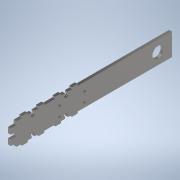
# Autodesk Inventor part: NeckFrame
Saved by Autodesk Inventor 2021 (Build 250183000, 183)
## iProperties
Created: 2021-03-05
Part Number: NeckFrame
Material: Steel, High Strength, Low Alloy
Document SubType Name: Modeling
Designer: M3rob
Density: 7.85 g/cm^3
Appearance: Steel - Polished
Mass: 7033.88 g
Surface Area: 1732.16 cm^2
Volume: 896.036 cm^3
Author: M3rob
Autodesk Inventor part; units mm, degrees
ref_plane "YZ Plane" through (0, 0, 0) normal (1, 0, 0) x (0, 1, 0)
ref_plane "XZ Plane" through (0, 0, 0) normal (0, 1, 0) x (-1, 0, 0)
ref_plane "XY Plane" through (0, 0, 0) normal (0, 0, 1) x (1, 0, 0)
sketch "Sketch1" plane through (0, 0, 0) normal (1, 0, 0) x (0, 1, 0)
  line L0 (50.8, 332.74) -> (34.925, 332.74)
  line L1 (-50.8, 332.74) -> (-50.8, -378.46)
  line L2 (-50.8, -378.46) -> (50.8, -378.46)
  line L3 (50.8, -378.46) -> (50.8, 53.34)
  circle A0 centre (0, -314.96) radius 25.4
  line L4 (50.8, 0) -> (-50.8, 0) construction
  line L5 (50.8, 307.34) -> (58.7375, 307.34)
  line L6 (58.7375, 307.34) -> (58.7375, 281.94)
  line L7 (58.7375, 281.94) -> (50.8, 281.94)
  line L8 (50.8, 281.94) -> (34.925, 281.94) construction
  line L9 (34.925, 281.94) -> (34.925, 307.34) construction
  line L10 (34.925, 307.34) -> (50.8, 307.34) construction
  line L11 (58.7375, 205.74) -> (50.8, 205.74)
  line L12 (58.7375, 231.14) -> (58.7375, 205.74)
  line L13 (50.8, 231.14) -> (58.7375, 231.14)
  line L14 (34.925, 231.14) -> (50.8, 231.14) construction
  line L15 (34.925, 205.74) -> (34.925, 231.14) construction
  line L16 (50.8, 205.74) -> (34.925, 205.74) construction
  line L17 (58.7375, 129.54) -> (50.8, 129.54)
  line L18 (58.7375, 154.94) -> (58.7375, 129.54)
  line L19 (50.8, 154.94) -> (58.7375, 154.94)
  line L20 (34.925, 154.94) -> (50.8, 154.94) construction
  line L21 (34.925, 129.54) -> (34.925, 154.94) construction
  line L22 (50.8, 129.54) -> (34.925, 129.54) construction
  line L23 (58.7375, 53.34) -> (50.8, 53.34)
  line L24 (58.7375, 78.74) -> (58.7375, 53.34)
  line L25 (50.8, 78.74) -> (58.7375, 78.74)
  line L26 (34.925, 78.74) -> (50.8, 78.74) construction
  line L27 (34.925, 53.34) -> (34.925, 78.74) construction
  line L28 (50.8, 53.34) -> (34.925, 53.34) construction
  line L29 (50.8, 281.94) -> (50.8, 307.34) construction
  line L30 (50.8, 307.34) -> (50.8, 332.74)
  line L31 (50.8, 231.14) -> (50.8, 249.7963)
  line L32 (50.8, 205.74) -> (50.8, 231.14) construction
  line L33 (50.8, 129.54) -> (50.8, 154.94) construction
  line L34 (50.8, 154.94) -> (50.8, 205.74)
  line L35 (50.8, 78.74) -> (50.8, 129.54)
  line L36 (50.8, 53.34) -> (50.8, 78.74) construction
  line L37 (50.8, 256.54) -> (30.1625, 256.54) construction
  line L38 (30.1625, 256.54) -> (30.1625, 249.7963)
  line L39 (30.1625, 249.7963) -> (33.3375, 249.7963)
  line L40 (33.3375, 249.7963) -> (33.3375, 247.015)
  line L41 (33.3375, 247.015) -> (41.275, 247.015)
  line L42 (41.275, 247.015) -> (41.275, 249.7963)
  line L43 (41.275, 249.7963) -> (50.8, 249.7963)
  line L44 (50.8, 263.2837) -> (41.275, 263.2837)
  line L45 (41.275, 263.2837) -> (41.275, 266.065)
  line L46 (41.275, 266.065) -> (33.3375, 266.065)
  line L47 (33.3375, 266.065) -> (33.3375, 263.2837)
  line L48 (33.3375, 263.2837) -> (30.1625, 263.2837)
  line L49 (30.1625, 263.2837) -> (30.1625, 256.54)
  line L50 (50.8, 249.7963) -> (50.8, 263.2837)
  line L51 (50.8, 263.2837) -> (50.8, 281.94)
  line L52 (-50.8, 307.34) -> (-58.7375, 307.34)
  line L53 (-58.7375, 307.34) -> (-58.7375, 281.94)
  line L54 (-58.7375, 281.94) -> (-50.8, 281.94)
  line L55 (-50.8, 307.34) -> (-34.964, 307.34) construction
  line L56 (-34.964, 307.34) -> (-34.964, 281.94) construction
  line L57 (-34.964, 281.94) -> (-50.8, 281.94) construction
  line L58 (-34.964, 231.14) -> (-34.964, 205.74) construction
  line L59 (-50.8, 231.14) -> (-34.964, 231.14) construction
  line L60 (-50.8, 231.14) -> (-58.7375, 231.14)
  line L61 (-58.7375, 231.14) -> (-58.7375, 205.74)
  line L62 (-58.7375, 205.74) -> (-50.8, 205.74)
  line L63 (-34.964, 205.74) -> (-50.8, 205.74) construction
  line L64 (-34.964, 154.94) -> (-34.964, 129.54) construction
  line L65 (-50.8, 154.94) -> (-34.964, 154.94) construction
  line L66 (-50.8, 154.94) -> (-58.7375, 154.94)
  line L67 (-58.7375, 154.94) -> (-58.7375, 129.54)
  line L68 (-58.7375, 129.54) -> (-50.8, 129.54)
  line L69 (-34.964, 129.54) -> (-50.8, 129.54) construction
  line L70 (-34.964, 78.74) -> (-34.964, 53.34) construction
  line L71 (-50.8, 78.74) -> (-34.964, 78.74) construction
  line L72 (-50.8, 78.74) -> (-58.7375, 78.74)
  line L73 (-58.7375, 78.74) -> (-58.7375, 53.34)
  line L74 (-58.7375, 53.34) -> (-50.8, 53.34)
  line L75 (-34.964, 53.34) -> (-50.8, 53.34) construction
  line L76 (0, 378.46) -> (0, 0) construction
  line L77 (-30.1625, 256.54) -> (-30.1625, 249.7963)
  line L78 (-30.1625, 249.7963) -> (-33.3375, 249.7963)
  line L79 (-33.3375, 249.7963) -> (-33.3375, 247.015)
  line L80 (-33.3375, 247.015) -> (-41.275, 247.015)
  line L81 (-41.275, 247.015) -> (-41.275, 249.7963)
  line L82 (-41.275, 249.7963) -> (-50.8, 249.7963)
  line L83 (-50.8, 263.2837) -> (-41.275, 263.2837)
  line L84 (-41.275, 263.2837) -> (-41.275, 266.065)
  line L85 (-41.275, 266.065) -> (-33.3375, 266.065)
  line L86 (-33.3375, 266.065) -> (-33.3375, 263.2837)
  line L87 (-33.3375, 263.2837) -> (-30.1625, 263.2837)
  line L88 (-30.1625, 263.2837) -> (-30.1625, 256.54)
  line L89 (-50.8, 249.7963) -> (-50.8, 263.2837)
  line L90 (-33.3375, 94.615) -> (-41.275, 94.615)
  line L91 (-41.275, 94.615) -> (-41.275, 97.3963)
  line L92 (-33.3375, 97.3963) -> (-33.3375, 94.615)
  line L93 (-41.275, 97.3963) -> (-50.8, 97.3963)
  line L94 (-30.1625, 97.3963) -> (-33.3375, 97.3963)
  line L95 (-30.1625, 104.14) -> (-30.1625, 97.3963)
  line L96 (-50.8, 97.3963) -> (-50.8, 110.8837)
  line L97 (-50.8, 110.8837) -> (-41.275, 110.8837)
  line L98 (-30.1625, 110.8837) -> (-30.1625, 104.14)
  line L99 (-41.275, 110.8837) -> (-41.275, 113.665)
  line L100 (-33.3375, 113.665) -> (-33.3375, 110.8837)
  line L101 (-41.275, 113.665) -> (-33.3375, 113.665)
  line L102 (-33.3375, 110.8837) -> (-30.1625, 110.8837)
  line L103 (50.8, 104.14) -> (30.1625, 104.14) construction
  line L104 (30.1625, 104.14) -> (30.1625, 97.3963)
  line L105 (30.1625, 97.3963) -> (33.3375, 97.3963)
  line L106 (33.3375, 97.3963) -> (33.3375, 94.615)
  line L107 (33.3375, 94.615) -> (41.275, 94.615)
  line L108 (41.275, 94.615) -> (41.275, 97.3963)
  line L109 (41.275, 97.3963) -> (50.8, 97.3963)
  line L110 (50.8, 110.8837) -> (41.275, 110.8837)
  line L111 (41.275, 110.8837) -> (41.275, 113.665)
  line L112 (41.275, 113.665) -> (33.3375, 113.665)
  line L113 (33.3375, 113.665) -> (33.3375, 110.8837)
  line L114 (33.3375, 110.8837) -> (30.1625, 110.8837)
  line L115 (30.1625, 110.8837) -> (30.1625, 104.14)
  line L116 (50.8, 97.3963) -> (50.8, 110.8837)
  line L117 (0, 0) -> (0, -378.46) construction
  line L118 (34.925, 332.74) -> (34.925, 358.14)
  line L119 (34.925, 358.14) -> (9.525, 358.14)
  line L120 (9.525, 358.14) -> (9.525, 332.74)
  line L121 (-9.525, 332.74) -> (-9.525, 358.14)
  line L122 (-9.525, 358.14) -> (-34.925, 358.14)
  line L123 (-34.925, 358.14) -> (-34.925, 332.74)
  line L124 (9.525, 345.44) -> (-9.525, 345.44) construction
  line L125 (34.925, 332.74) -> (9.525, 332.74) construction
  line L126 (9.525, 332.74) -> (-9.525, 332.74)
  line L127 (-9.525, 332.74) -> (-34.925, 332.74) construction
  line L128 (-34.925, 332.74) -> (-50.8, 332.74)
  line L129 (34.925, 25.4) -> (9.525, 25.4)
  line L130 (9.525, 25.4) -> (9.525, 12.7)
  line L131 (9.525, 12.7) -> (34.925, 12.7)
  line L132 (34.925, 12.7) -> (34.925, 25.4)
  line L133 (-9.525, 25.4) -> (-34.925, 25.4)
  line L134 (-34.925, 25.4) -> (-34.925, 12.7)
  line L135 (-34.925, 12.7) -> (-9.525, 12.7)
  line L136 (-9.525, 12.7) -> (-9.525, 25.4)
  line L137 (-9.525, 139.7) -> (-34.925, 139.7)
  line L138 (34.925, 139.7) -> (9.525, 139.7)
  line L139 (9.525, 127) -> (34.925, 127)
  line L140 (34.925, 127) -> (34.925, 139.7)
  line L141 (9.525, 139.7) -> (9.525, 127)
  line L142 (-9.525, 127) -> (-9.525, 139.7)
  line L143 (-34.925, 127) -> (-9.525, 127)
  line L144 (-34.925, 139.7) -> (-34.925, 127)
  point P0 (50.8, 0)
  point P1 (0, 345.44)
  dimension "d0" = 711.2
  dimension "d1" = 101.6
  dimension "d4" = 50.8
  dimension "d5" = 63.5
  dimension "d6" = 332.74
  dimension "d7" = 25.4
  dimension "d8" = 7.9375
  dimension "d11" = 76.2
  dimension "d16" = 13.4874
  dimension "d17" = 9.525
  dimension "d18" = 7.9375
  dimension "d19" = 3.175
  dimension "d20" = 19.05
  dimension "d23" = 76.2
  dimension "d33" = 152.4
  dimension "d35" = 19.05
  dimension "d36" = 25.4
  dimension "d37" = 25.4
  dimension "d38" = 12.7
  dimension "d39" = 25.4
  dimension "d40" = 391.16
  dimension "d41" = 19.05
  dimension "d44" = 114.3
  constraints: 290 end point, 45 perpendicular, 42 point on line, 21 parallel, 15 symmetric about line, 12 horizontal, 9 equal length, 7 midpoint, 7 vertical, 3 vertical alignment, 2 horizontal alignment, 1 centre point, 1 collinear, 144 other
  measures "d0" distance of L2.end L0.start
  measures "d1" distance of L0.start L1.start
  measures "d4" diameter of A0
  measures "d5" distance from line of L2 A0.centre
  measures "d6" distance between parallel lines of L0 L4
  measures "d7" distance of L5.end L6.end
  measures "d8" distance of L6.end L7.end
  measures "d11" distance of L6.end L11.start
  measures "d16" distance between parallel lines of L44 L43
  measures "d17" distance of L31.end L42.end
  measures "d18" distance of L40.end L41.end
  measures "d19" distance of L38.end L39.end
  measures "d20" distance between parallel lines of L46 L41
  measures "d23" distance of L55.end L58.start
  measures "d33" distance of L80.end L90.end
  measures "d35" distance between parallel lines of L121 L120
  measures "d36" distance of L118.end L119.end
  measures "d37" distance of L0.end L118.end
  measures "d38" distance of L131.end L129.start
  measures "d39" distance of L130.end L131.end
  measures "d40" distance between parallel lines of L2 L131
  measures "d41" distance between parallel lines of L136 L130
  measures "d44" distance of L129.end L138.end
extrude "Extrusion1" add sketch "Sketch1" along normal mid plane 12.7 contours L30 L5 L6 L7 L51 L44 L45 L46 L47 L48 L49 L38 L39 L40 L41 L42 L43 L31 L13 L12 L11 L34 L19 L18 L17 L35 L110 L111 L112 L113 L114 L115 L104 L105 L106 L107 L108 L109 L25 L24 L23 L3 L2 L1 L93 L91 L90 L92 L94 L95 L98 L102 L100 L101 L99 L97 L82 L81 L80 L79 L78 L77 L88 L87 L86 L85 L84 L83 L128 L123 L122 L121 L126 L120 L119 L118 L0 | L1 L54 L53 L52 | L1 L62 L61 L60 | L1 L68 L67 L66 | L1 L74 L73 L72
sketch "Sketch2" plane through (6.35, 0, 0) normal (1, 0, 0) x (0, 0, -1)
  circle A0 centre (314.96, 0) radius 25.4 projected
  circle A1 centre (-279.4, 0.127) radius 101.6 construction
  line L0 (-327.1798, -89.5371) -> (135.7856, -336.2403) construction
  line L1 (66.4469, 0) -> (66.4469, -299.2914) construction
  line L2 (-22.4531, 0) -> (-22.4531, -251.9187) construction
  line L3 (-53.34, -50.8) -> (378.46, -50.8) construction
  arc A2 (314.9383, -50.8) -> (66.4469, -299.2914) centre (314.9383, -299.2914) ccw
  line L4 (-53.34, 50.8) -> (378.46, 50.8) construction
  arc A3 (66.5748, 299.3975) -> (314.96, 50.8) centre (315.0662, 299.2914) ccw
  line L5 (-279.4, 0.127) -> (314.96, 0) construction
  line L6 (66.5748, 299.3975) -> (-22.3454, 252.0629)
  line L7 (-22.4531, -251.9187) -> (66.4469, -299.2914)
  arc A4 (-142.24, 50.8) -> (-22.3454, 252.0629) centre (-251.3834, 252.1607) ccw
  arc A5 (-22.4531, -251.9187) -> (-141.9023, -50.8) centre (-251.4911, -251.9187) ccw
  arc A6 (22.0169, -181.8764) -> (-53.34, -50.8) centre (-251.4911, -251.9187) ccw
  arc A7 (120.4101, -50.8) -> (22.0169, -181.8764) centre (314.9383, -299.2914) ccw
  arc A8 (22.1147, 163.2651) -> (108.7273, 50.8) centre (315.0662, 299.2914) ccw
  arc A9 (-46.0604, 50.8) -> (22.1147, 163.2651) centre (-251.3834, 252.1607) ccw
  line L8 (21.9969, -275.605) -> (22.0558, 0.0626) construction
  line L9 (22.1147, 50.8) -> (22.1147, 275.7302) construction
  line L10 (-142.24, 50.8) -> (-46.0604, 50.8)
  line L11 (-141.9023, -50.8) -> (-53.34, -50.8)
  line L12 (108.7273, 50.8) -> (314.96, 50.8)
  line L13 (314.9383, -50.8) -> (120.4101, -50.8)
  point P0 (0, 0)
  dimension "d49" = 762
  dimension "d50" = 88.9
  dimension "d51" = 457.2
  constraints: 24 end point, 16 point on circle, 12 point on line, 8 centre point, 4 concentric, 4 midpoint, 4 perpendicular, 4 tangent, 2 horizontal alignment, 2 parallel, 2 symmetric about line, 1 coincident, 1 collinear, 1 horizontal, 1 vertical alignment, 9 other
  measures "d50" distance between parallel lines of L2 L1
  measures "d51" distance of L12.end L10.start
extrude "Extrusion2" [suppressed]
body "Solid1"
body "Solid2"
